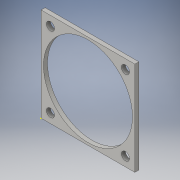
# Autodesk Inventor part: FanLip
Saved by Autodesk Inventor 2016 (Build 200138000, 138)
## iProperties
Created: 2016-08-18
Part Number: FanLip
Material: Generic
Document SubType Name: Modeling
Designer: yash
Density: 1 g/cm^3
Appearance: Default
Author: yash
Autodesk Inventor part; units mm, degrees
ref_plane "YZ Plane" through (0, 0, 0) normal (1, 0, 0) x (0, 1, 0)
ref_plane "XZ Plane" through (0, 0, 0) normal (0, 1, 0) x (-1, 0, 0)
ref_plane "XY Plane" through (0, 0, 0) normal (0, 0, 1) x (1, 0, 0)
sketch "Sketch1" plane through (0, 0, 0) normal (0, 0, 1) x (1, 0, 0)
  line L0 (0, 0) -> (40, 0)
  line L1 (40, 0) -> (40, 40)
  line L2 (40, 40) -> (0, 40)
  line L3 (0, 40) -> (0, 0)
  circle A0 centre (20, 20) radius 19
  point P0 (20, 0)
  point P1 (40, 20)
  dimension "d0" = 40
  dimension "d1" = 40
  dimension "d2" = 38
  constraints: 8 end point, 2 midpoint, 2 parallel, 1 centre point, 1 horizontal, 1 horizontal alignment, 1 perpendicular, 1 vertical alignment
  measures "d0" distance of L2.end L1.end
  measures "d1" distance of L1.end L0.end
  measures "d2" diameter of A0
extrude "Extrusion1" add sketch "Sketch1" along normal blind 1.7272
sketch "Sketch2" plane through (0, 0, 1.7272) normal (0, 0, 1) x (1, 0, 0)
  point P0 (0, 0)
sketch "Sketch3" plane through (0, 0, 1.7272) normal (0, 0, 1) x (1, 0, 0)
  line L0 (0, 40) -> (0, 0) construction
  line L1 (0, 0) -> (40, 0) construction
  point P0 (4, 36)
  point P1 (36, 36)
  point P2 (36, 4)
  point P3 (4, 4)
  point P4 (20, 20)
  dimension "d5" = 32
  dimension "d6" = 32
  dimension "d7" = 32
  dimension "d8" = 20
  dimension "d9" = 20
  dimension "d10" = 16
  dimension "d11" = 16
  constraints: 2 horizontal alignment, 1 vertical alignment
  measures "d5" distance of point (4, 36) point (36, 36)
  measures "d6" distance of point (4, 4) point (4, 36)
  measures "d7" distance of point (36, 4) point (4, 4)
  measures "d8" distance from line of L0 point (20, 20)
  measures "d9" distance from line of L1 point (20, 20)
  measures "d10" horizontal distance of point (4, 36) point (20, 20)
  measures "d11" horizontal distance of point (4, 36) point (20, 20)
hole "Hole1" at (36, 36, 1.7272) at (4, 36, 1.7272) at (4, 4, 1.7272) at (36, 4, 1.7272) direction (0, 0, -1) diameter 3.5 end through all
body "Solid1"
